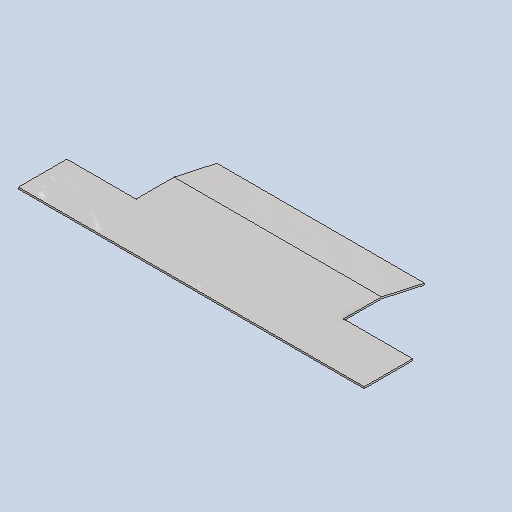
# Autodesk Inventor part: tyl
Saved by Autodesk Inventor 2023 (Build 270158000, 158)
## iProperties
Created: 2023-07-07
Part Number: tyl
Material: Stal miękka, spawana
Document SubType Name: Modeling
Designer: Kamil
Density: 7.85 g/cm^3
Appearance: Spawane — stal miękka
Author: Kamil
Autodesk Inventor part; units mm, degrees
ref_plane "YZ Plane" through (0, 0, 0) normal (1, 0, 0) x (0, 1, 0)
ref_plane "XZ Plane" through (0, 0, 0) normal (0, 1, 0) x (-1, 0, 0)
ref_plane "XY Plane" through (0, 0, 0) normal (0, 0, 1) x (1, 0, 0)
sketch "Szkic1" plane through (0, 0, 0) normal (0, 1, 0) x (-1, 0, 0)
  line L0 (0, 0) -> (-100, 0)
  line L1 (-100, 0) -> (-100, -14)
  line L2 (-100, -14) -> (0, -14)
  line L3 (0, -14) -> (0, 0)
  dimension "d0" = 100
  dimension "d1" = 14
  constraints: 8 end point, 2 parallel, 1 horizontal, 1 perpendicular
  measures "d0" distance of L2.end L1.end
  measures "d1" distance of L1.end L0.end
extrude "Wyciągnięcie proste1" add sketch "Szkic1" along normal blind 0.5
sketch "Szkic2" plane through (0, 0.5, 0) normal (0, 1, 0) x (1, 0, 0)
  line L0 (100, 14) -> (0, 14) projected
  line L1 (80, 14) -> (20, 14)
  line L2 (20, 14) -> (20, 25)
  line L3 (20, 25) -> (80, 25)
  line L4 (80, 25) -> (80, 14)
  point P0 (0, 0)
  point P1 (50, 14)
  point P2 (50, 14)
  point P3 (50, 14)
  dimension "d4" = 60
  dimension "d5" = 11
  constraints: 8 end point, 4 midpoint, 2 parallel, 1 coincident, 1 horizontal, 1 perpendicular
  measures "d4" distance of L2.end L3.end
  measures "d5" distance of L1.end L2.end
extrude "Wyciągnięcie proste2" add sketch "Szkic2" against normal blind 0.5
sketch "Szkic3" plane through (80, 0.5, -14) normal (1, 0, 0) x (0, 0, -1)
  line L0 (0, 0) -> (11, 0) projected
  line L1 (0, -0.5) -> (0, 0) projected
  line L2 (11, -0.5) -> (0, -0.5) projected
  line L3 (11, 0) -> (11, -0.5) projected
  line L4 (11, 0) -> (23.4078, -2.7462)
  line L5 (11, -0.5) -> (23.3023, -3.2228)
  line L6 (23.3023, -3.2228) -> (23.4078, -2.7462)
  point P0 (-14, -0.5)
  dimension "d8" = 167.52
  dimension "d9" = 12.6
  constraints: 6 end point, 1 parallel, 1 perpendicular
  measures "d8" angle of L5 L2
  measures "d9" distance of L2.start L5.end
extrude "Wyciągnięcie proste3" add sketch "Szkic3" against normal up to surface (60 mm away) contours L4 L6 L5 L3
